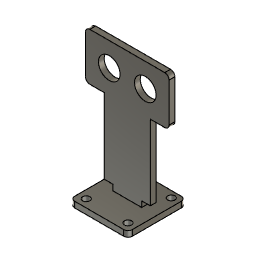
US-senzor holder (Autodesk Fusion 360 design; units mm, degrees)
Autodesk Fusion 360 part; units mm, degrees
sketch "Sketch1" plane through (0, 0, 0) normal (0, 0, 1) x (1, 0, 0)
  line L0 (-16, -42.5) -> (-16, 9.5)
  line L1 (16, 9.5) -> (16, -42.5)
  line L2 (-29, 12.5) -> (-29, 39.5)
  line L3 (-26, 42.5) -> (26, 42.5)
  line L4 (29, 39.5) -> (29, 12.5)
  line L5 (26, 9.5) -> (16, 9.5)
  line L6 (-16, 9.5) -> (-26, 9.5)
  circle A0 centre (12.5, 26) radius 7.5
  line L7 (0, 100) -> (0, -110) construction
  circle A1 centre (-12.5, 26) radius 7.5
  arc A2 (-26, 42.5) -> (-29, 39.5) centre (-26, 39.5) ccw
  arc A3 (29, 39.5) -> (26, 42.5) centre (26, 39.5) ccw
  arc A4 (26, 9.5) -> (29, 12.5) centre (26, 12.5) ccw
  arc A5 (-29, 12.5) -> (-26, 9.5) centre (-26, 12.5) ccw
  line L8 (-10, -42.5) -> (-10, -50.5)
  line L9 (-10, -50.5) -> (10, -50.5)
  line L10 (10, -50.5) -> (10, -42.5)
  line L11 (16, -42.5) -> (10, -42.5)
  line L12 (-10, -42.5) -> (-16, -42.5)
  point P0 (-29, 42.5)
  point P1 (29, 42.5)
  point P2 (0, 26)
  dimension "d3" = 58
  dimension "d7" = 32
  dimension "d8" = 52
  dimension "d9" = 85
  dimension "d13" = 3
  dimension "d14" = 3
  dimension "d15" = 25
  dimension "d16" = 16.5
  dimension "d18" = 8
  dimension "d19" = 20
  constraint horizontal L11
  constraint perpendicular L0 L11
  constraint parallel L0 L1
  constraint horizontal L5
  constraint perpendicular L2 L5
  constraint parallel L3 L5
  constraint parallel L2 L4
  constraint coincident L0.end L5
  constraint collinear L5 L6
  constraint perpendicular L7 L11
  constraint symmetric A0 L7 A1
  constraint coincident P0 L2
  constraint coincident P0 L3
  constraint tangent L2 A2
  constraint tangent L3 A2
  constraint coincident P1 L3
  constraint coincident P1 L4
  constraint tangent L3 A3
  constraint tangent L4 A3
  constraint tangent L4 A4
  constraint tangent L5 A4
  constraint equal A3 A4
  constraint tangent L2 A5
  constraint tangent L6 A5
  constraint equal A3 A5
  constraint perpendicular L8 L11
  constraint perpendicular L8 L9
  constraint perpendicular L10 L11
  constraint collinear L11 L12
  measures "d3" distance of P0 P1
  measures "d7" distance of L0 L1
  measures "d8" distance of L5 L11
  measures "d9" distance of L3 L11
  measures "d13" radius of A2
  measures "d14" radius of A3
  measures "d15" distance of A0.centre A1.centre
  measures "d16" distance of L3 A0.centre
  measures "d18" distance of L8.start L8.end
  measures "d19" distance of L8.end L9.end
extrude "Extrude1" add sketch "Sketch1" along normal blind 4 makes body 1
move_body "Move1" bodies 1 to x (1, 0, 0) y (0, 0, 1) z (0, -1, 0) at (0, -50.5, 50.5)
sketch "Sketch2" plane through (0, 0, 0) normal (0, 0, 1) x (1, 0, 0)
  line L0 (120, -20) -> (80, -20)
  line L1 (80, -20) -> (80, 20)
  line L2 (80, 20) -> (120, 20)
  line L3 (120, 20) -> (120, -20)
  line L4 (110, -0.5) -> (90, -0.5)
  line L5 (90, -0.5) -> (90, 3.5)
  line L6 (90, 3.5) -> (110, 3.5)
  line L7 (110, 3.5) -> (110, -0.5)
  line L8 (110, -0.5) -> (90, 3.5) construction
  line L9 (90, -0.5) -> (110, 3.5) construction
  circle A0 centre (114.5, 15.5) radius 2.5
  line L10 (100, 40) -> (100, -30) construction
  line L11 (60, 0) -> (140, 0) construction
  circle A1 centre (114.5, -14.5) radius 2.5
  circle A2 centre (85.5, 15.5) radius 2.5
  circle A3 centre (85.5, -14.5) radius 2.5
  point P0 (100, 1.5)
  point P1 (100, 1.5)
  dimension "d22" = 40
  dimension "d23" = 40
  dimension "d24" = 4
  dimension "d27" = 5
  dimension "d36" = 30
  dimension "d37" = 12
  constraint horizontal L0
  constraint perpendicular L0 L1
  constraint parallel L0 L2
  constraint parallel L1 L3
  constraint horizontal L4
  constraint perpendicular L4 L5
  constraint parallel L4 L6
  constraint parallel L5 L7
  constraint coincident L8 P1
  constraint coincident L9 P1
  constraint coincident P1 P0
  constraint perpendicular L4 L10
  constraint perpendicular L3 L11
  constraint symmetric A0 L10 A2
  constraint symmetric L10 A1 A3
  measures "d22" distance of L1.end L2.end
  measures "d23" distance of L0.end L1.end
  measures "d24" distance of L4.end L5.end
  measures "d27" diameter of A0
  measures "d36" distance of A0.centre A1.centre
  measures "d37" distance of L6 A0.centre
extrude "Extrude2" add sketch "Sketch2" along normal blind 4 separate body makes body 2
fillet "Fillet1" radius 3 4 edges at (120, -20, 2) (120, 20, 2) (80, 20, 2) (80, -20, 2) on bodies 2
copy_body "Body->Comp1" bodies 2 removing the originals makes body 3 in component "Component"
component "Component" placed x (1, 0, 0) y (0, 1, 0) z (0, 0, 1) at (-100, -54, 0)
